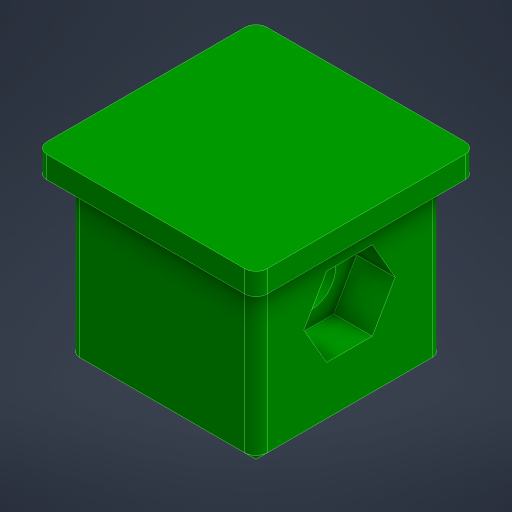
# Autodesk Inventor part: holder
Saved by Autodesk Inventor 2024 (Build 280153000, 153)
## iProperties
Created: 2023-05-14
Part Number: holder
Material: Типовые
Document SubType Name: Modeling
Designer: user
Density: 1 g/cm^3
Appearance: По умолчанию
Author: user
Autodesk Inventor part; units mm, degrees
ref_plane "YZ Plane" through (0, 0, 0) normal (1, 0, 0) x (0, 1, 0)
ref_plane "XZ Plane" through (0, 0, 0) normal (0, 1, 0) x (-1, 0, 0)
sketch "Эскиз1" plane through (0, 0, 0) normal (0, 0, 1) x (1, 0, 0)
  line L0 (0, 0) -> (17, 0)
  line L1 (17, 0) -> (17, 17)
  line L2 (17, 17) -> (0, 17)
  line L3 (0, 17) -> (0, 0)
  dimension "d0" = 17
  dimension "d1" = 17
  constraints: 8 end point, 2 parallel, 1 horizontal, 1 perpendicular
  measures "d0" distance of L1.end L2.end
  measures "d1" distance of L0.end L1.end
extrude "Выдавливание1" add sketch "Эскиз1" against normal blind 15
sketch "Эскиз2" plane through (17, 0, 0) normal (1, 0, 0) x (0, 0, -1)
  line L0 (6, 4.3431) -> (2.4, 6.4215)
  line L1 (2.4, 6.4215) -> (2.4, 10.5785)
  line L2 (2.4, 10.5785) -> (6, 12.6569)
  line L3 (6, 12.6569) -> (9.6, 10.5785)
  line L4 (9.6, 10.5785) -> (9.6, 6.4215)
  line L5 (9.6, 6.4215) -> (6, 4.3431)
  line L6 (0, 17) -> (15, 17) projected
  line L7 (15, 17) -> (15, 0) projected
  point P0 (0, 0)
  point P1 (6, 8.5)
  point P2 (15, 8.5)
  point P3 (15, 8.5)
  dimension "d4" = 7.2
  dimension "d21" = 6
  constraints: 12 end point, 2 midpoint, 1 horizontal alignment, 1 vertical, 13 other
  measures "d4" distance of L3.end L1.end
  measures "d21" horizontal distance of point (0, 0) point (6, 8.5)
extrude "Выдавливание2" cut sketch "Эскиз2" against normal blind 3.5
ref_plane "РабПлоскость1" through (8.5, 0, 0) normal (1, 0, 0) x (0, 0, -1)
mirror "Зеркальное отражение1" about plane through (8.5, 0, 0) normal (1, 0, 0) of "Выдавливание2"
shell "Оболочка1" thickness 3.5 removed faces 1 at (5.6667, 11.3333, -15)
sketch "Эскиз3" plane through (0, 0, 0) normal (0, 0, 1) x (1, 0, 0)
  line L0 (-1.5, -1.5) -> (18.5, -1.5)
  line L1 (18.5, -1.5) -> (18.5, 18.5)
  line L2 (18.5, 18.5) -> (-1.5, 18.5)
  line L3 (-1.5, 18.5) -> (-1.5, -1.5)
  line L4 (0, 0) -> (17, 0) projected
  line L5 (17, 0) -> (17, 17) projected
  point P0 (8.5, 0)
  point P1 (8.5, -1.5)
  point P2 (17, 8.5)
  point P3 (18.5, 8.5)
  dimension "d8" = 20
  constraints: 8 end point, 4 midpoint, 2 parallel, 2 perpendicular, 1 horizontal, 1 horizontal alignment, 1 vertical alignment
  measures "d8" distance of L1.end L2.end
extrude "Выдавливание3" add sketch "Эскиз3" along normal blind 2
fillet "Сопряжение1" radius 1 8 edges at (-1.5, -1.5, 1) (0, 0, -7.5) (18.5, -1.5, 1) (17, 0, -7.5) (18.5, 18.5, 1) (17, 17, -7.5) (0, 17, -7.5) (-1.5, 18.5, 1)
chamfer "Фаска1" distance 1 angle 45 8 edges at (0, 8.5, -15) (0.2929, 16.7071, -15) (8.5, 17, -15) (16.7071, 16.7071, -15) (17, 8.5, -15) (16.7071, 0.2929, -15) (8.5, 0, -15) (0.2929, 0.2929, -15)
sketch "Эскиз4" plane through (13.5, 0, 0) normal (1, 0, 0) x (0, 0, -1)
  circle A0 centre (6, 8.5) radius 2.25
  line L0 (9.6, 10.5785) -> (9.6, 6.4215) projected
  point P0 (0, 0)
  point P1 (6, 4.3431)
  point P2 (9.6, 8.5)
  dimension "d15" = 4.5
  constraints: 1 centre point, 1 horizontal alignment, 1 midpoint, 1 vertical alignment
  measures "d15" diameter of A0
extrude "Выдавливание4" cut sketch "Эскиз4" against normal through all
equation "\"d1\" = d0"
